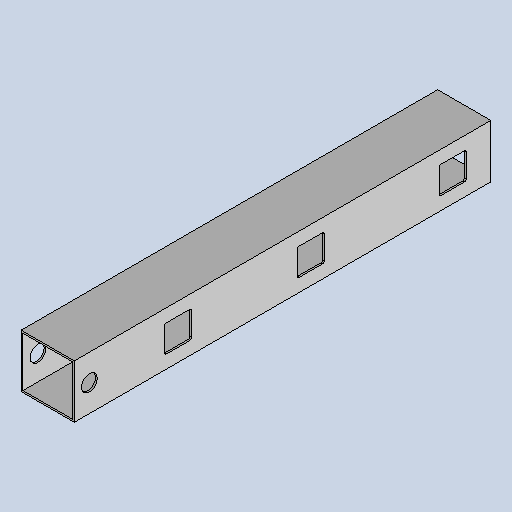
# Autodesk Inventor part: PNS 753 FDS 1200 colector tube !!
Saved by Autodesk Inventor 2025.1 (Build 291241020, 241B)
## iProperties
Created: 2025-06-24
Part Number: PNS 753 FDS 1200 colector tube !!
Material: Stainless Steel
Description: DIE16(5)|\ 90°|corrY -___°|X_____|bom___
Document SubType Name: Modeling
Designer: user
Mass: 1762.25 g
Surface Area: 2283.33 cm^2
Volume: 220.281 cm^3
Density: 8 g/cm^3
Sheet Metal Width: 0.000 mm
Sheet Metal Length: 0.000 mm
Sheet Metal Area: 0.000 mm^2
Appearance: Default
Sheet Metal Rule: AISI304 2mm Die16
Author: user
Autodesk Inventor part; units mm, degrees
ref_plane "YZ Plane" through (0, 0, 0) normal (1, 0, 0) x (0, 1, 0)
ref_plane "XZ Plane" through (0, 0, 0) normal (0, 1, 0) x (-1, 0, 0)
ref_plane "XY Plane" through (0, 0, 0) normal (0, 0, 1) x (1, 0, 0)
sketch "Sketch9" plane through (0, 0, 0) normal (0, 1, 0) x (-1, 0, 0)
  line L0 (30, 30) -> (-30, 30)
  line L1 (-30, 30) -> (-30, -30)
  line L2 (-30, -30) -> (30, -30)
  line L3 (30, -30) -> (30, 30)
  line L4 (30, 30) -> (-30, -30) construction
  line L5 (-30, 30) -> (30, -30) construction
  line L6 (-28, 28) -> (28, 28)
  line L7 (28, 28) -> (28, -28)
  line L8 (28, -28) -> (-28, -28)
  line L9 (-28, -28) -> (-28, 28)
  point P0 (0, 0)
  dimension "d172" = 60
  dimension "d173" = 60
  dimension "d174" = 2
  constraints: 20 end point, 4 parallel, 2 midpoint, 2 perpendicular, 1 horizontal, 3 other
  measures "d172" distance of L2.end L1.end
  measures "d173" distance of L0.end L1.end
  measures "d174" distance between parallel lines of L0 L6
extrude "Extrusion3" add sketch "Sketch9" against normal blind 470
sketch "Sketch10" plane through (0, 0, 0) normal (1, 0, 0) x (0, 1, 0)
  line L0 (0, 30) -> (0, -30) construction
  line L1 (0, 30) -> (-470, 30) construction
  line L2 (-470, -30) -> (-470, 30) construction
  line L3 (0, -30) -> (-470, -30) construction
  line L4 (-58.25, 15.25) -> (-27.75, 15.25)
  line L5 (-27.75, 15.25) -> (-27.75, -15.25)
  line L6 (-27.75, -15.25) -> (-58.25, -15.25)
  line L7 (-58.25, -15.25) -> (-58.25, 15.25)
  line L8 (-58.25, 15.25) -> (-27.75, -15.25) construction
  line L9 (-27.75, 15.25) -> (-58.25, -15.25) construction
  line L10 (-218.25, 15.25) -> (-187.75, 15.25)
  line L11 (-187.75, 15.25) -> (-187.75, -15.25)
  line L12 (-187.75, -15.25) -> (-218.25, -15.25)
  line L13 (-218.25, -15.25) -> (-218.25, 15.25)
  line L14 (-218.25, 15.25) -> (-187.75, -15.25) construction
  line L15 (-187.75, 15.25) -> (-218.25, -15.25) construction
  line L16 (-368.25, 15.25) -> (-337.75, 15.25)
  line L17 (-337.75, 15.25) -> (-337.75, -15.25)
  line L18 (-337.75, -15.25) -> (-368.25, -15.25)
  line L19 (-368.25, -15.25) -> (-368.25, 15.25)
  line L20 (-368.25, 15.25) -> (-337.75, -15.25) construction
  line L21 (-337.75, 15.25) -> (-368.25, -15.25) construction
  circle A0 centre (-453, 0) radius 9
  line L22 (0, 0) -> (47, 0)
  point P0 (-43, 0)
  point P1 (-203, 0)
  point P2 (-353, 0)
  dimension "d177" = 30.5
  dimension "d178" = 30.5
  dimension "d181" = 47
  dimension "d182" = 90
  dimension "d183" = 250
  dimension "d184" = 400
  dimension "d185" = 500
  dimension "d186" = 18
  constraints: 38 end point, 7 midpoint, 6 parallel, 4 horizontal, 4 horizontal alignment, 3 equal length, 3 perpendicular, 1 centre point, 1 point on line
  measures "d177" distance of L4.start L4.end
  measures "d178" distance of L4.end L5.end
  measures "d181" distance of L22.start L22.end
  measures "d182" distance of point (-43, 0) L22.end
  measures "d183" distance of point (-203, 0) L22.end
  measures "d184" distance of L22.end point (-353, 0)
  measures "d185" distance of L22.end A0.centre
  measures "d186" diameter of A0
extrude "Extrusion4" cut sketch "Sketch10" along normal through all both and the other way through all
sketch "Sketch11" plane through (30, 0, 30) normal (1, 0, 0) x (0, 0, -1)
  line L0 (45.25, -218.25) -> (14.75, -218.25) projected
  line L1 (14.75, -218.25) -> (14.75, -187.75) projected
  line L2 (14.75, -187.75) -> (45.25, -187.75) projected
  line L3 (45.25, -187.75) -> (45.25, -218.25) projected
  circle A0 centre (30, -453) radius 9 projected
  line L4 (45.25, -58.25) -> (14.75, -58.25) projected
  line L5 (14.75, -58.25) -> (14.75, -27.75) projected
  line L6 (14.75, -27.75) -> (45.25, -27.75) projected
  line L7 (45.25, -27.75) -> (45.25, -58.25) projected
  line L8 (45.25, -368.25) -> (14.75, -368.25) projected
  line L9 (14.75, -368.25) -> (14.75, -337.75) projected
  line L10 (14.75, -337.75) -> (45.25, -337.75) projected
  line L11 (45.25, -337.75) -> (45.25, -368.25) projected
  line L12 (0, 0) -> (60, 0) projected
  line L13 (0, 0) -> (0, -470) projected
  line L14 (60, -470) -> (0, -470) projected
  line L15 (60, 0) -> (60, -470) projected
  line L16 (45.25, -27.75) -> (14.75, -58.25)
  line L17 (45.25, -187.75) -> (14.75, -218.25)
  line L18 (45.25, -337.75) -> (14.75, -368.25)
  point P0 (30, 0)
  constraints: 6 end point, 2 parallel, 1 point on line
sketch "Sketch13" plane through (-30, 0, -30) normal (-1, 0, 0) x (0, 0, 1)
  line L0 (45.25, -218.25) -> (14.75, -218.25) projected
  line L1 (14.75, -218.25) -> (14.75, -187.75) projected
  line L2 (14.75, -187.75) -> (45.25, -187.75) projected
  line L3 (45.25, -187.75) -> (45.25, -218.25) projected
  circle A0 centre (30, -453) radius 9 projected
  line L4 (45.25, -58.25) -> (14.75, -58.25) projected
  line L5 (14.75, -58.25) -> (14.75, -27.75) projected
  line L6 (14.75, -27.75) -> (45.25, -27.75) projected
  line L7 (45.25, -27.75) -> (45.25, -58.25) projected
  line L8 (45.25, -368.25) -> (14.75, -368.25) projected
  line L9 (14.75, -368.25) -> (14.75, -337.75) projected
  line L10 (14.75, -337.75) -> (45.25, -337.75) projected
  line L11 (45.25, -337.75) -> (45.25, -368.25) projected
  line L12 (0, 0) -> (60, 0) projected
  line L13 (0, 0) -> (0, -470) projected
  line L14 (60, -470) -> (0, -470) projected
  line L15 (60, 0) -> (60, -470) projected
  line L16 (14.75, -58.25) -> (45.25, -27.75)
  line L17 (14.75, -218.25) -> (45.25, -187.75)
  line L18 (14.75, -368.25) -> (45.25, -337.75)
  point P0 (30, 0)
  constraints: 6 end point, 2 parallel
fillet "Fillet1" radius 2 24 edges at (29, -337.75, -15.25) (29, -337.75, 15.25) (29, -368.25, 15.25) (29, -368.25, -15.25) (29, -218.25, -15.25) (29, -218.25, 15.25) (29, -187.75, 15.25) (29, -187.75, -15.25) (29, -58.25, 15.25) (29, -27.75, 15.25) (29, -27.75, -15.25) (29, -58.25, -15.25) (-29, -58.25, 15.25) (-29, -27.75, 15.25) (-29, -27.75, -15.25) (-29, -58.25, -15.25) (-29, -187.75, 15.25) (-29, -218.25, 15.25) (-29, -218.25, -15.25) (-29, -187.75, -15.25) (-29, -337.75, 15.25) (-29, -368.25, 15.25) (-29, -337.75, -15.25) (-29, -368.25, -15.25)
body "Solid4"
